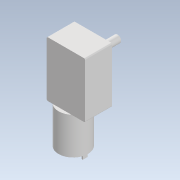
# Autodesk Inventor part: motor_dc_12v_90d
Saved by Autodesk Inventor 2020.2 (Build 242310000, 310)
## iProperties
Created: 2020-04-13
Part Number: motor_dc_12v_90d
Material: Generic
Document SubType Name: Modeling
Designer: Bardo91
Density: 1 g/cm^3
Appearance: Default
Author: Bardo91
Autodesk Inventor part; units mm, degrees
ref_plane "YZ Plane" through (0, 0, 0) normal (1, 0, 0) x (0, 1, 0)
ref_plane "XZ Plane" through (0, 0, 0) normal (0, 1, 0) x (-1, 0, 0)
ref_plane "XY Plane" through (0, 0, 0) normal (0, 0, 1) x (1, 0, 0)
sketch "Sketch1" plane through (0, 0, 0) normal (0, 0, 1) x (1, 0, 0)
  line L0 (0, 0) -> (15, 0)
  line L1 (16, 1) -> (16, 45)
  line L2 (15, 46) -> (-15, 46)
  line L3 (-16, 45) -> (-16, 1)
  line L4 (-15, 0) -> (16, 0)
  arc A0 (-15, 46) -> (-16, 45) centre (-15, 45) ccw
  arc A1 (16, 45) -> (15, 46) centre (15, 45) ccw
  arc A2 (15, 0) -> (16, 1) centre (15, 1) ccw
  arc A3 (-16, 1) -> (-15, 0) centre (-15, 1) ccw
  point P0 (16, 46)
  point P1 (-16, 46)
  dimension "d0" = 16
  dimension "d1" = 46
  dimension "d2" = 32
  dimension "d3" = 1
  constraints: 10 end point, 8 point on circle, 8 tangent, 6 point on line, 4 centre point, 3 equal radius, 2 horizontal, 1 collinear, 1 perpendicular, 1 vertical
  measures "d0" distance of L0.start L4.end
  measures "d1" distance of L4.end point (16, 46)
  measures "d2" distance of point (16, 46) point (-16, 46)
  measures "d3" radius of A0
extrude "Extrusion1" add sketch "Sketch1" along normal blind 22.5
sketch "Sketch2" plane through (0, 0, 0) normal (0, 0, -1) x (-1, 0, 0)
  line L0 (0, 0) -> (-10, 0)
  line L1 (15, 0) -> (-15, 0) projected
  line L2 (-10, 0) -> (-10, 7)
  line L3 (-10, 7) -> (-10, 40)
  circle A0 centre (-10, 7) radius 3.7
  circle A1 centre (-10, 40) radius 3.7
  line L4 (-10, 40) -> (8, 40)
  line L5 (-10, 7) -> (8, 7)
  circle A2 centre (8, 7) radius 3.7
  circle A3 centre (8, 40) radius 3.7
  line L6 (-15, 46) -> (15, 46) projected
  line L7 (0, 46) -> (0, 31)
  circle A4 centre (0, 31) radius 6
  dimension "d6" = 10
  dimension "d7" = 7
  dimension "d8" = 33
  dimension "d9" = 7.4
  dimension "d10" = 7.4
  dimension "d11" = 18
  dimension "d12" = 18
  dimension "d13" = 7.4
  dimension "d14" = 7.4
  dimension "d23" = 15
  dimension "d24" = 12
  constraints: 12 end point, 5 centre point, 5 coincident, 2 horizontal, 2 point on line, 1 midpoint, 1 perpendicular, 1 vertical
  measures "d6" distance of L0.start L0.end
  measures "d7" distance of L0.end L2.end
  measures "d8" distance of L2.end L3.end
  measures "d9" diameter of A0
  measures "d10" diameter of A1
  measures "d11" distance of L4.start L4.end
  measures "d12" distance of L5.start L5.end
  measures "d13" diameter of A2
  measures "d14" diameter of A3
  measures "d23" distance of L7.start L7.end
  measures "d24" diameter of A4
extrude "Extrusion2" add sketch "Sketch2" along normal blind 2
sketch "Sketch3" plane through (10, 7, -2) normal (0, 0, -1) x (-1, 0, 0)
  circle A0 centre (0, 0) radius 3.7 projected
  circle A1 centre (0, 0) radius 1.5
  circle A2 centre (0, 33) radius 3.7 projected
  circle A3 centre (0, 33) radius 1.5
  circle A4 centre (18, 33) radius 3.7 projected
  circle A5 centre (18, 33) radius 1.5
  circle A6 centre (18, 0) radius 3.7 projected
  circle A7 centre (18, 0) radius 1.5
  point P0 (10, -7)
  dimension "d17" = 3
  dimension "d18" = 3
  dimension "d19" = 3
  dimension "d20" = 3
  constraints: 4 centre point, 4 coincident
  measures "d17" diameter of A1
  measures "d18" diameter of A3
  measures "d19" diameter of A5
  measures "d20" diameter of A7
extrude "Extrusion3" cut sketch "Sketch3" against normal blind 3 contours A1 | A3 | A5 | A7
sketch "Sketch4" plane through (0, 31, -2) normal (0, 0, -1) x (-1, 0, 0)
  circle A0 centre (0, 0) radius 6 projected
  circle A1 centre (0, 0) radius 3
  point P0 (0, -31)
  dimension "d25" = 6
  constraints: 1 centre point, 1 coincident
  measures "d25" diameter of A1
extrude "Extrusion4" add sketch "Sketch4" along normal blind 18.5 contours A1
sketch "Sketch5" plane through (0, 31, -20.5) normal (0, 0, -1) x (-1, 0, 0)
  circle A0 centre (0, 0) radius 3 projected
  line L0 (0, 3) -> (0, -2.4)
  line L1 (0, -2.4) -> (-1.8, -2.4)
  line L2 (0, -2.4) -> (1.8, -2.4)
  point P0 (0, -31)
  dimension "d28" = 5.4
  constraints: 6 end point, 3 point on circle, 1 perpendicular, 1 point on line, 1 vertical
  measures "d28" distance of L0.start L0.end
extrude "Extrusion5" cut sketch "Sketch5" against normal blind 10 contours A0 L1 L2
sketch "Sketch6" plane through (-15, 0, 0) normal (0, -1, 0) x (1, 0, 0)
  circle A0 centre (11.8, 13.2) radius 12.2
  line L0 (-1, 0) -> (-1, 22.5) projected
  line L1 (0, 0) -> (30, 0) projected
  point P0 (15, 0)
  dimension "d31" = 24.4
  dimension "d40" = 13.2
  dimension "d41" = 12.8
  constraints: 1 centre point
  measures "d31" diameter of A0
  measures "d40" distance from line of L1 A0.centre
  measures "d41" distance from line of A0.centre L0
extrude "Extrusion6" add sketch "Sketch6" along normal blind 30.8
sketch "Sketch7" plane through (-3.2, -30.8, 13.2) normal (0, -1, 0) x (1, 0, 0)
  line L0 (0, 0) -> (10, 0)
  line L1 (10, 0) -> (10, -2)
  line L2 (10, -2) -> (10, 2)
  line L3 (10, 2) -> (9, 2)
  line L4 (9, 2) -> (9, -2)
  line L5 (9, -2) -> (10, -2)
  line L6 (0, 0) -> (0, -2)
  line L7 (0, 0) -> (-10, 0)
  line L8 (-10, 0) -> (-10, -2)
  line L9 (-10, -2) -> (-10, 2)
  line L10 (-10, 2) -> (-9, 2)
  line L11 (-9, 2) -> (-9, -2)
  line L12 (-9, -2) -> (-10, -2)
  point P0 (3.2, -13.2)
  dimension "d34" = 10
  dimension "d35" = 2
  dimension "d36" = 4
  dimension "d37" = 1
  constraints: 26 end point, 5 perpendicular, 5 symmetric about line, 3 point on line, 1 horizontal
  measures "d34" distance of L0.start L0.end
  measures "d35" distance of L0.end L1.end
  measures "d36" distance of L1.end L2.end
  measures "d37" distance of L2.end L3.end
extrude "Extrusion7" add sketch "Sketch7" along normal blind 4.2
equation "\"d0\" = 0.5 * d2"
body "Solid1"
